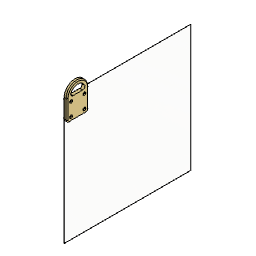
Backpack Bracket (Autodesk Fusion 360 design; units mm, degrees)
Autodesk Fusion 360 part; units mm, degrees
sketch "Sketch1" plane through (0, 0, 0) normal (1, 0, 0) x (0, 1, 0) in component "Sheet"
  line L0 (0, 0) -> (200, 0)
  line L1 (200, 0) -> (200, -200)
  line L2 (200, -200) -> (0, -200)
  line L3 (0, -200) -> (0, 0)
  dimension "d1" = 200
  dimension "d2" = 200
  constraint horizontal L0
  constraint vertical L1
  constraint horizontal L2
  constraint vertical L3
  constraint coincident L0.start L3.end
  measures "d1" distance of L0.start L0.end
  measures "d2" distance of L0.start L2.end
extrude "Extrude1" add sketch "Sketch1" along normal blind 0.2 makes body 1 in component "Sheet"
sketch "Sketch1 (2)" plane through (0, 0, 0) normal (-1, 0, 0) x (0, -1, 0) in component "Inside Bracket"
  line L0 (-200, -200) -> (0, -200)
  line L1 (0, -200) -> (0, 0)
  line L2 (0, 0) -> (-200, 0)
  line L3 (-200, 0) -> (-200, -200)
  line L4 (-4, 0) -> (-30, 0)
  line L5 (-34, -4) -> (-34, -30)
  line L6 (-30, -34) -> (-4, -34)
  line L7 (0, -30) -> (0, -4)
  arc A0 (-30, 0) -> (-34, -4) centre (-30, -4) ccw
  arc A1 (0, -4) -> (-4, 0) centre (-4, -4) ccw
  arc A2 (-4, -34) -> (0, -30) centre (-4, -30) ccw
  arc A3 (-34, -30) -> (-30, -34) centre (-30, -30) ccw
  line L8 (-17, 0) -> (-17, -34) construction
  line L9 (-34, -17) -> (0, -17) construction
  line L10 (-6.5, -6.5) -> (-27.5, -6.5) construction
  line L11 (-27.5, -6.5) -> (-27.5, -27.5) construction
  line L12 (-27.5, -27.5) -> (-6.5, -27.5) construction
  line L13 (-6.5, -27.5) -> (-6.5, -6.5) construction
  line L14 (-6.5, -6.5) -> (-27.5, -27.5) construction
  line L15 (-27.5, -6.5) -> (-6.5, -27.5) construction
  circle A4 centre (-27.5, -6.5) radius 1.075
  circle A5 centre (-27.5, -6.5) radius 2.6
  circle A6 centre (-6.5, -6.5) radius 1.075
  circle A7 centre (-6.5, -6.5) radius 2.6
  circle A8 centre (-27.5, -27.5) radius 2.6
  circle A9 centre (-27.5, -27.5) radius 1.075
  circle A10 centre (-6.5, -27.5) radius 1.075
  circle A11 centre (-6.5, -27.5) radius 2.6
  point P0 (-34, 0)
  point P1 (0, -34)
  point P2 (-17, -17)
  dimension "d5" = 34
  dimension "d6" = 34
  dimension "d7" = 4
  dimension "d8" = 21
  dimension "d9" = 21
  dimension "d15" = 2.15
  dimension "d16" = 5.2
  dimension "d17" = 2.15
  dimension "d18" = 5.2
  dimension "d19" = 5.2
  dimension "d20" = 2.15
  dimension "d21" = 2.15
  dimension "d22" = 5.2
  constraint horizontal L4
  constraint vertical L5
  constraint horizontal L6
  constraint vertical L7
  constraint coincident L1.end L2.start
  constraint coincident P0 L5
  constraint coincident P0 L4
  constraint tangent L5 A0
  constraint tangent L4 A0
  constraint coincident L1.end L4
  constraint coincident L1.end L7
  constraint tangent L4 A1
  constraint tangent L7 A1
  constraint equal A0 A1
  constraint coincident P1 L7
  constraint coincident P1 L6
  constraint tangent L7 A2
  constraint tangent L6 A2
  constraint equal A0 A2
  constraint tangent L6 A3
  constraint tangent L5 A3
  constraint equal A0 A3
  constraint midpoint L4 L8.start
  constraint midpoint L6 L8.end
  constraint midpoint L5 L9.start
  constraint midpoint L7 L9.end
  constraint horizontal L10
  constraint perpendicular L10 L11
  constraint parallel L10 L12
  constraint parallel L11 L13
  constraint coincident L14 P2
  constraint coincident L15 P2
  constraint midpoint L8 P2
  constraint coincident L10.end L11.start
  constraint concentric A4 A5
  constraint coincident L10.start L13.end
  constraint concentric A6 A7
  constraint coincident L11.end L12.start
  constraint concentric A8 A9
  constraint coincident L12.end L13.start
  constraint concentric A10 A11
  measures "d5" distance of L1.end P0
  measures "d6" distance of L1.end P1
  measures "d7" radius of A0
  measures "d8" distance of L11.end L12.end
  measures "d9" distance of L10.end L11.end
  measures "d15" diameter of A4
  measures "d16" diameter of A5
  measures "d17" diameter of A6
  measures "d18" diameter of A7
  measures "d19" diameter of A8
  measures "d20" diameter of A9
  measures "d21" diameter of A10
  measures "d22" diameter of A11
extrude "Extrude1'" add sketch "Sketch1 (2)" along normal blind 2.7 separate body contours L1 L2 L4 L5 L6 L7 A0 A1 A2 A3 makes body 2 in component "Inside Bracket"
extrude "Extrude2" add sketch "Sketch1 (2)" along normal blind 1 contours A5 | A7 | A8 | A11 bodies 2 in component "Inside Bracket"
fillet "Fillet1" radius 4 8 edges at (-2.7, 32.8284, -32.8284) (-2.7, 17, -34) (-2.7, 1.1716, -32.8284) (-2.7, 0, -17) (-2.7, 1.1716, -1.1716) (-2.7, 17, 0) (-2.7, 32.8284, -1.1716) (-2.7, 34, -17) on bodies 2 in component "Inside Bracket"
sketch "Sketch1 (3)" plane through (0.2, 0, 0) normal (1, 0, 0) x (0, 1, 0) in component "Outside Bracket"
  line L0 (0, -200) -> (200, -200)
  line L1 (200, -200) -> (200, 0)
  line L2 (200, 0) -> (0, 0)
  line L3 (0, 0) -> (0, -200)
  circle A0 centre (6.5, -6.5) radius 1.075
  circle A1 centre (27.5, -27.5) radius 1.075
  circle A2 centre (6.5, -27.5) radius 1.075
  circle A3 centre (6.5, -6.5) radius 1.075
  circle A4 centre (27.5, -6.5) radius 1.075
  arc A5 (30, -34) -> (34, -30) centre (30, -30) ccw
  line L4 (34, -30) -> (34, -4)
  arc A6 (34, -4) -> (30, 0) centre (30, -4) ccw
  line L5 (30, 0) -> (4, 0)
  arc A7 (4, 0) -> (0, -4) centre (4, -4) ccw
  line L6 (0, -4) -> (0, -30)
  arc A8 (0, -30) -> (4, -34) centre (4, -30) ccw
  line L7 (4, -34) -> (30, -34)
  line L8 (17, 0) -> (17, -34) construction
  line L9 (0, -17) -> (34, -17) construction
  line L10 (34, 0) -> (0, 0)
  line L11 (0, 0) -> (0, -34)
  line L12 (0, -34) -> (34, -34) construction
  line L13 (34, -34) -> (34, 0)
  line L14 (34, 0) -> (0, -34) construction
  line L15 (0, 0) -> (34, -34) construction
  line L16 (34, -4) -> (34, -30) construction
  circle A9 centre (17, 0) radius 17
  circle A10 centre (17, 0) radius 12
  line L17 (8.55, -5.3164) -> (6.5, -4.1329)
  line L18 (6.5, -4.1329) -> (4.45, -5.3164)
  line L19 (4.45, -5.3164) -> (4.45, -7.6836)
  line L20 (4.45, -7.6836) -> (6.5, -8.8671)
  line L21 (6.5, -8.8671) -> (8.55, -7.6836)
  line L22 (8.55, -7.6836) -> (8.55, -5.3164)
  line L23 (29.55, -5.3164) -> (29.55, -7.6836)
  line L24 (29.55, -7.6836) -> (27.5, -8.8671)
  line L25 (27.5, -8.8671) -> (25.45, -7.6836)
  line L26 (25.45, -7.6836) -> (25.45, -5.3164)
  line L27 (25.45, -5.3164) -> (27.5, -4.1329)
  line L28 (27.5, -4.1329) -> (29.55, -5.3164)
  line L29 (25.45, -28.6836) -> (27.5, -29.8671)
  line L30 (27.5, -29.8671) -> (29.55, -28.6836)
  line L31 (29.55, -28.6836) -> (29.55, -26.3164)
  line L32 (29.55, -26.3164) -> (27.5, -25.1329)
  line L33 (27.5, -25.1329) -> (25.45, -26.3164)
  line L34 (25.45, -26.3164) -> (25.45, -28.6836)
  line L35 (8.55, -28.6836) -> (6.5, -29.8671)
  line L36 (6.5, -29.8671) -> (4.45, -28.6836)
  line L37 (4.45, -28.6836) -> (4.45, -26.3164)
  line L38 (4.45, -26.3164) -> (6.5, -25.1329)
  line L39 (8.55, -26.3164) -> (8.55, -28.6836)
  line L40 (6.5, -25.1329) -> (8.55, -26.3164)
  point P0 (17, -17)
  point P1 (6.5, -6.5)
  dimension "d29" = 5
  dimension "d30" = 2.05
  constraint midpoint L5 L8.start
  constraint midpoint L7 L8.end
  constraint midpoint L6 L9.start
  constraint midpoint L4 L9.end
  constraint horizontal L10
  constraint perpendicular L10 L11
  constraint parallel L10 L12
  constraint parallel L11 L13
  constraint coincident L14 P0
  constraint coincident L15 P0
  constraint coincident L5 L10.start
  constraint midpoint L9 P0
  constraint collinear L13 L16
  constraint coincident L8.start A9.centre
  constraint coincident L10.start A9
  constraint concentric A9 A10
  constraint coincident P1 A0.centre
  constraint vertical L22
  constraint symmetric L8 L17.start L26.end
  constraint symmetric L8 L17.end L27.end
  constraint symmetric L8 L18.end L23.start
  constraint symmetric L8 L19.end L23.end
  constraint symmetric L8 L20.end L24.end
  constraint symmetric L8 L21.end L25.end
  constraint symmetric L9 L17.start L35.start
  constraint symmetric L9 L17.end L35.end
  constraint symmetric L9 L18.end L36.end
  constraint symmetric L9 L19.end L37.end
  constraint symmetric L9 L20.end L38.end
  constraint symmetric L9 L21.end L39.start
  constraint symmetric L9 L23.start L30.end
  constraint symmetric L9 L23.end L31.end
  constraint symmetric L9 L24.end L32.end
  constraint symmetric L9 L25.end L33.end
  constraint symmetric L9 L26.end L29.start
  constraint symmetric L9 L27.end L29.end
  measures "d29" distance of A9 A10
  measures "d30" distance of P1 L22
extrude "Extrude1''" add sketch "Sketch1 (3)" along normal blind 4.5 separate body contours L3 A5 L4 A6 A7 L6 A8 L7 L11 L13 A9 | L2 A6 L10 A9 | L2 L5 L10 A9 A10 | A6 L13 A9 | L3 A7 L11 A9 | L2 A6 L5 A7 L10 A9 A10 L18 L19 L20 L21 L23 L24 L25 L28 | L2 A7 L10 A9 | L2 L5 L10 A10 L17 L18 L21 L22 L25 L26 L27 L28 makes body 3 in component "Outside Bracket"
extrude "Extrude2'" add sketch "Sketch1 (3)" along normal blind 2.5 contours A4 A10 L23 L24 L25 L28 | A4 A10 L25 L26 L27 L28 | A0 A3 A10 L17 L18 L21 L22 | A0 A3 A10 L18 L19 L20 L21 | L29 L30 L31 L32 L33 L34 | L35 L36 L37 L38 L39 L40 bodies 3 in component "Outside Bracket"
fillet "Fillet1'" radius 3.5 2 edges at (2.45, 5, 0) (2.45, 29, 0) on bodies 3 in component "Outside Bracket"
fillet "Fillet2" radius 1.5 6 edges at (4.7, 1.1716, -32.8284) (4.7, 17, -34) (4.7, 32.8284, -32.8284) (4.7, 34, -15) (4.7, 17, 17) (4.7, 0, -15) on bodies 3 in component "Outside Bracket"
component "Sheet" placed x (1, 0, 0) y (0, 1, 0) z (0, 0, 1) at (0, 0, 0)
component "Inside Bracket" placed x (1, 0, 0) y (0, 1, 0) z (0, 0, 1) at (0, 0, 0)
component "Outside Bracket" placed x (1, 0, 0) y (0, 1, 0) z (0, 0, 1) at (0, 0, 0)
equation "d8 = d9"
equation "screw_diam = 2.15 mm"
equation "washer_diam = 5.2 mm"
equation "nut_diam = 4.1 mm"
equation "d15 = screw_diam"
equation "d16 = washer_diam"
equation "d17 = screw_diam"
equation "d18 = washer_diam"
equation "d19 = washer_diam"
equation "d20 = screw_diam"
equation "d21 = screw_diam"
equation "d22 = washer_diam"
equation "d30 = ( 4.1 / 2 ) * 1 mm"
